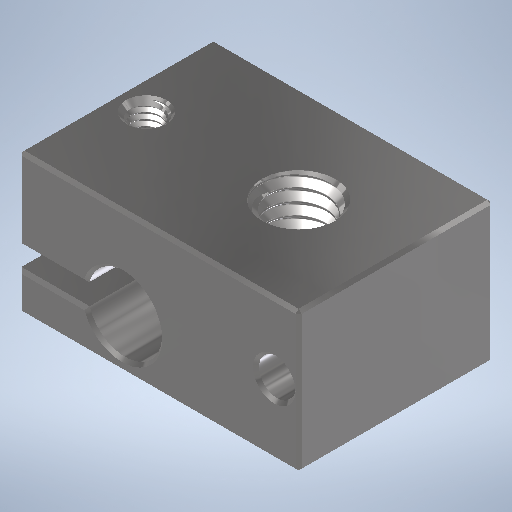
# Autodesk Inventor part: E3D-v6 Heater Block for Sensor Cartridges
Saved by Autodesk Inventor 2025.2 (Build 292293000, 293)
## iProperties
Created: 2018-03-24
Part Number: E3D-v6 Heater Block for Sensor Cartridges
Material: Aluminum 7075
Document SubType Name: Modeling
Designer: Samppa Turunen
Density: 2.81 g/cm^3
Appearance: Semi-Polished
Author: Samppa Turunen
Autodesk Inventor part; units mm, degrees
ref_plane "YZ Plane" through (0, 0, 0) normal (1, 0, 0) x (0, 1, 0)
ref_plane "XZ Plane" through (0, 0, 0) normal (0, 1, 0) x (-1, 0, 0)
ref_plane "XY Plane" through (0, 0, 0) normal (0, 0, 1) x (1, 0, 0)
sketch "Sketch1" plane through (0, 0, 0) normal (0, 1, 0) x (-1, 0, 0)
  line L0 (11.5, 8) -> (-11.5, 8)
  line L1 (-11.5, 8) -> (-11.5, -8)
  line L2 (-11.5, -8) -> (11.5, -8)
  line L3 (11.5, -8) -> (11.5, 8)
  line L4 (11.5, 8) -> (-11.5, -8) construction
  line L5 (-11.5, 8) -> (11.5, -8) construction
  point P0 (0, 0)
  dimension "d0" = 23
  dimension "d1" = 16
  constraints: 12 end point, 2 midpoint, 2 parallel, 1 horizontal, 1 perpendicular
  measures "d0" distance of L0.start L0.end
  measures "d1" distance of L1.end L0.end
extrude "Extrusion1" add sketch "Sketch1" along normal blind 11.5
sketch "Sketch2" plane through (0, 11.5, 0) normal (0, 1, 0) x (1, 0, 0)
  circle A0 centre (-9, 0) radius 1.5
  circle A1 centre (3.5, 0) radius 3
  point P0 (0, 0)
  dimension "d5" = 3
  dimension "d6" = 6
  constraints: 2 centre point
  measures "d5" diameter of A0
  measures "d6" diameter of A1
extrude "Extrusion2" cut sketch "Sketch2" against normal through all
sketch "Sketch3" plane through (-11.5, 0, 8) normal (0, 0, 1) x (1, 0, 0)
  circle A0 centre (21, 5.75) radius 1.5
  arc A1 (5.5872, 3.1) -> (5.5571, 4.7969) centre (8.5013, 4.0004) ccw
  line L0 (0, 3.1) -> (5.5872, 3.1)
  line L1 (0, 4.7969) -> (5.5571, 4.7969)
  line L2 (0, 3.1) -> (0, 4.7969)
  point P0 (11.5, 0)
  dimension "d9" = 3
  dimension "d10" = 6.1
  constraints: 6 end point, 2 centre point, 2 point on circle, 1 perpendicular
  measures "d9" diameter of A0
  measures "d10" diameter of A1
extrude "Extrusion3" cut sketch "Sketch3" along normal through all both and the other way through all
sketch "Sketch4" plane through (0, 0, 0) normal (0, -1, 0) x (1, 0, 0)
  circle A0 centre (9.5, 0) radius 1.5
  point P0 (0, 0)
  dimension "d13" = 3
  constraints: 1 centre point
  measures "d13" diameter of A0
extrude "Extrusion4" cut sketch "Sketch4" against normal up to next
sketch "Sketch6" plane through (3.5, 0, 0) normal (-1, 0, 0) x (0, 0, 1)
  line L0 (3.0474, 0) -> (3.0474, 11.5)
  line L1 (2.3474, 10.8) -> (2.3474, 0.7)
  line L2 (0, -2.3) -> (0, 13.8) projected
  line L3 (3.0474, 11.5) -> (2.3474, 10.8)
  line L4 (3.0474, 0) -> (2.3474, 0.7)
  dimension "d40" = 0.7
  constraints: 8 end point, 1 vertical
  measures "d40" distance between parallel lines of L0 L1
revolve "Revolution1" add sketch "Sketch6" angle 360 about axis through (3.5, 0, 0) along (0, 1, 0) separate body
sketch "Sketch5" plane through (3.5, 0, 3) normal (1, 0, 0) x (0, 1, 0)
  line L0 (-0.5925, -0.0535) -> (-0.5001, -0.0535) construction
  line L1 (0.0923, -0.5994) -> (-0.0001, -0.7595) construction
  line L2 (-1.0001, -0.7595) -> (-1.0925, -0.5994) construction
  line L3 (-0.4077, -0.0535) -> (-0.5001, 0.1066) construction
  line L4 (-0.5001, 0.1066) -> (-0.5925, -0.0535) construction
  line L5 (-1.0001, -0.7595) -> (-0.9077, -0.5994) construction
  line L6 (-0.4077, -0.0535) -> (-0.0925, -0.5994)
  line L7 (-1.0925, -0.5994) -> (-0.9077, -0.5994) construction
  arc A0 (-1.0925, -0.5994) -> (-1.0001, -0.6528) centre (-1.0001, -0.546) ccw construction
  line L8 (0.0923, -0.5994) -> (-0.0925, -0.5994) construction
  line L9 (-1.0001, -0.7595) -> (-1.0001, -0.5994) construction
  line L10 (-0.0001, -0.7595) -> (-0.0001, -0.5994) construction
  line L11 (-0.5001, 0.1066) -> (-0.5001, -0.0002) construction
  line L12 (-1.0001, -0.6528) -> (-0.0001, -0.6528)
  arc A1 (-1.0001, -0.6528) -> (-0.9077, -0.5994) centre (-1.0001, -0.546) ccw
  line L13 (-0.0925, -0.5994) -> (-0.0001, -0.7595) construction
  line L14 (-0.9077, -0.5994) -> (-0.5925, -0.0535)
  line L15 (-0.0001, -0.0002) -> (-0.0001, 0.0177)
  line L16 (-0.0001, 0.0177) -> (-0.0001, -0.0002)
  line L17 (-0.0001, -0.0002) -> (0.0334, -0.0002)
  arc A2 (-0.0925, -0.5994) -> (-0.0001, -0.6528) centre (-0.0001, -0.546) ccw
  arc A3 (-0.0001, -0.6528) -> (0.0923, -0.5994) centre (-0.0001, -0.546) ccw construction
  arc A4 (-0.5001, -0.0002) -> (-0.5925, -0.0535) centre (-0.5001, -0.1069) ccw
  arc A5 (-0.4077, -0.0535) -> (-0.5001, -0.0002) centre (-0.5001, -0.1069) ccw
  line L18 (-0.5001, -0.0002) -> (-0.5001, -0.0535) construction
  line L19 (-0.5001, -0.0535) -> (-0.4077, -0.0535) construction
  dimension "d22" = 60
  dimension "d23" = 0.1601
  dimension "d24" = 0.1601
  dimension "Sketch5_ThreadOffset" = 0
  dimension "Sketch5_MajorRadius" = 0.6526
  dimension "d27" = 1
  dimension "Sketch5_MinorRadius" = 0
  constraints: 40 end point, 12 point on circle, 10 parallel, 8 tangent, 6 centre point, 6 collinear, 2 midpoint, 2 point on line, 1 horizontal, 1 perpendicular, 3 other
  measures "d22" angle of L6 L14
  measures "d23" distance of L3.end L0.end
  measures "d24" distance of L1.end L10.end
  measures "Sketch5_ThreadOffset" distance between parallel lines of L15 L10
  measures "Sketch5_MajorRadius" distance from line of L12 L15.start
  measures "d27" distance from line of L1.end L9
  measures "Sketch5_MinorRadius" distance edge to line of A5 L17
coil "Coil1" sketch "Sketch5" operation cut axis through (3.5, 0, 0) along (0, 1, 0) pitch 1.001 turns 13.486513 hand right bodies 2
sketch "Sketch8" plane through (-9, 4.7969, 0) normal (-1, 0, 0) x (0, 0, 1)
  line L0 (1.6737, 0) -> (1.6737, 6.7031)
  line L1 (1.1737, 6.2031) -> (1.1737, 0)
  line L2 (1.1737, 0) -> (1.6737, 0)
  line L3 (0, -1.3406) -> (0, 8.0438) projected
  line L4 (1.6737, 6.7031) -> (1.1737, 6.2031)
  dimension "d60" = 0.5
  dimension "d62" = 45
  constraints: 8 end point, 1 vertical
  measures "d60" distance between parallel lines of L0 L1
  measures "d62" angle of L0 L4
revolve "Revolution2" add sketch "Sketch8" angle 360 about axis through (-9, 4.7969, 0) along (0, 1, 0) separate body
chamfer "Chamfer2" distance 0.047 angle 45 2 edges at (3.5, 0, -3.0474) (3.5, 11.5, -3.0474)
sketch "Sketch7" plane through (-9, 4.7969, 1.5) normal (1, 0, 0) x (0, 1, 0)
  line L0 (-0.2963, -0.0268) -> (-0.2501, -0.0268) construction
  line L1 (0.0461, -0.2998) -> (-0.0001, -0.3798) construction
  line L2 (-0.5001, -0.3798) -> (-0.5463, -0.2998) construction
  line L3 (-0.2039, -0.0268) -> (-0.2501, 0.0532) construction
  line L4 (-0.2501, 0.0532) -> (-0.2963, -0.0268) construction
  line L5 (-0.5001, -0.3798) -> (-0.4539, -0.2998) construction
  line L6 (-0.2039, -0.0268) -> (-0.0463, -0.2998)
  line L7 (-0.5463, -0.2998) -> (-0.4539, -0.2998) construction
  arc A0 (-0.5463, -0.2998) -> (-0.5001, -0.3265) centre (-0.5001, -0.2731) ccw construction
  line L8 (0.0461, -0.2998) -> (-0.0463, -0.2998) construction
  line L9 (-0.5001, -0.3798) -> (-0.5001, -0.2998) construction
  line L10 (-0.0001, -0.3798) -> (-0.0001, -0.2998) construction
  line L11 (-0.2501, 0.0532) -> (-0.2501, -0.0002) construction
  line L12 (-0.5001, -0.3265) -> (-0.0001, -0.3265)
  arc A1 (-0.5001, -0.3265) -> (-0.4539, -0.2998) centre (-0.5001, -0.2731) ccw
  line L13 (-0.0463, -0.2998) -> (-0.0001, -0.3798) construction
  line L14 (-0.4539, -0.2998) -> (-0.2963, -0.0268)
  line L15 (-0.0001, -0.0002) -> (-0.0001, 0.0177)
  line L16 (-0.0001, 0.0177) -> (-0.0001, -0.0002)
  line L17 (-0.0001, -0.0002) -> (0.0334, -0.0002)
  arc A2 (-0.0463, -0.2998) -> (-0.0001, -0.3265) centre (-0.0001, -0.2731) ccw
  arc A3 (-0.0001, -0.3265) -> (0.0461, -0.2998) centre (-0.0001, -0.2731) ccw construction
  arc A4 (-0.2501, -0.0002) -> (-0.2963, -0.0268) centre (-0.2501, -0.0535) ccw
  arc A5 (-0.2039, -0.0268) -> (-0.2501, -0.0002) centre (-0.2501, -0.0535) ccw
  line L18 (-0.2501, -0.0002) -> (-0.2501, -0.0268) construction
  line L19 (-0.2501, -0.0268) -> (-0.2039, -0.0268) construction
  dimension "d42" = 60
  dimension "d43" = 0.08
  dimension "d44" = 0.08
  dimension "Sketch7_ThreadOffset" = 0
  dimension "Sketch7_MajorRadius" = 0.3263
  dimension "d47" = 0.5
  dimension "Sketch7_MinorRadius" = 0
  constraints: 40 end point, 12 point on circle, 10 parallel, 8 tangent, 6 centre point, 6 collinear, 2 midpoint, 2 point on line, 1 horizontal, 1 perpendicular, 3 other
  measures "d42" angle of L6 L14
  measures "d43" distance of L3.end L0.end
  measures "d44" distance of L1.end L10.end
  measures "Sketch7_ThreadOffset" distance between parallel lines of L15 L10
  measures "Sketch7_MajorRadius" distance from line of L12 L15.start
  measures "d47" distance from line of L1.end L9
  measures "Sketch7_MinorRadius" distance edge to line of A5 L17
coil "Coil2" sketch "Sketch7" operation cut axis through (-9, 4.7969, 0) along (0, 1, 0) pitch 0.5005 turns 15.390901 hand right bodies 3
sketch "Sketch10" plane through (9.5, 5.75, 0) normal (1, 0, 0) x (0, 0, 1)
  line L0 (1.6737, 0) -> (1.6737, 5.75)
  line L1 (1.1737, 5.25) -> (1.1737, 0)
  line L2 (1.1737, 0) -> (1.6737, 0)
  line L3 (0, -1.15) -> (0, 6.9) projected
  line L4 (1.6737, 5.75) -> (1.1737, 5.25)
  line L5 (1.6737, 5.75) -> (2.3808, 5.75) construction
  line L6 (-1.5, 5.75) -> (1.5, 5.75) projected
  dimension "d81" = 0.5
  dimension "d82" = 135
  dimension "d92" = 5.75
  constraints: 10 end point, 1 equal length, 1 horizontal, 1 vertical
  measures "d81" distance between parallel lines of L0 L1
  measures "d82" angle of L4 L5
  measures "d92" distance between parallel lines of L6 L2
revolve "Revolution3" add sketch "Sketch10" angle 360 about axis through (9.5, 5.75, 0) along (0, -1, 0) separate body
sketch "Sketch13" plane through (-11.5, 0, 8) normal (0, 0, 1) x (1, 0, 0)
  circle A0 centre (21, 5.75) radius 1.5 projected
  circle A1 centre (21, 5.75) radius 1.5
  line L0 (22.5, 0) -> (22.5, 5.75) projected
  point P0 (11.5, 0)
  constraints: 1 centre point, 1 coincident, 1 horizontal alignment, 1 tangent
extrude "Extrusion5" cut sketch "Sketch13" against normal through all bodies 1 2 4
sketch "Sketch9" plane through (9.5, 5.75, 1.5) normal (-1, 0, 0) x (0, -1, 0)
  line L0 (-0.2963, -0.0268) -> (-0.2501, -0.0268) construction
  line L1 (0.0461, -0.2998) -> (-0.0001, -0.3798) construction
  line L2 (-0.5001, -0.3798) -> (-0.5463, -0.2998) construction
  line L3 (-0.2039, -0.0268) -> (-0.2501, 0.0532) construction
  line L4 (-0.2501, 0.0532) -> (-0.2963, -0.0268) construction
  line L5 (-0.5001, -0.3798) -> (-0.4539, -0.2998) construction
  line L6 (-0.2039, -0.0268) -> (-0.0463, -0.2998)
  line L7 (-0.5463, -0.2998) -> (-0.4539, -0.2998) construction
  arc A0 (-0.5463, -0.2998) -> (-0.5001, -0.3265) centre (-0.5001, -0.2731) ccw construction
  line L8 (0.0461, -0.2998) -> (-0.0463, -0.2998) construction
  line L9 (-0.5001, -0.3798) -> (-0.5001, -0.2998) construction
  line L10 (-0.0001, -0.3798) -> (-0.0001, -0.2998) construction
  line L11 (-0.2501, 0.0532) -> (-0.2501, -0.0002) construction
  line L12 (-0.5001, -0.3265) -> (-0.0001, -0.3265)
  arc A1 (-0.5001, -0.3265) -> (-0.4539, -0.2998) centre (-0.5001, -0.2731) ccw
  line L13 (-0.0463, -0.2998) -> (-0.0001, -0.3798) construction
  line L14 (-0.4539, -0.2998) -> (-0.2963, -0.0268)
  line L15 (-0.0001, -0.0002) -> (-0.0001, 0.0177)
  line L16 (-0.0001, 0.0177) -> (-0.0001, -0.0002)
  line L17 (-0.0001, -0.0002) -> (0.0334, -0.0002)
  arc A2 (-0.0463, -0.2998) -> (-0.0001, -0.3265) centre (-0.0001, -0.2731) ccw
  arc A3 (-0.0001, -0.3265) -> (0.0461, -0.2998) centre (-0.0001, -0.2731) ccw construction
  arc A4 (-0.2501, -0.0002) -> (-0.2963, -0.0268) centre (-0.2501, -0.0535) ccw
  arc A5 (-0.2039, -0.0268) -> (-0.2501, -0.0002) centre (-0.2501, -0.0535) ccw
  line L18 (-0.2501, -0.0002) -> (-0.2501, -0.0268) construction
  line L19 (-0.2501, -0.0268) -> (-0.2039, -0.0268) construction
  dimension "d63" = 60
  dimension "d64" = 0.08
  dimension "d65" = 0.08
  dimension "Sketch9_ThreadOffset" = 0
  dimension "Sketch9_MajorRadius" = 0.3263
  dimension "d68" = 0.5
  dimension "Sketch9_MinorRadius" = 0
  constraints: 40 end point, 12 point on circle, 10 parallel, 8 tangent, 6 centre point, 6 collinear, 2 midpoint, 2 point on line, 1 horizontal, 1 perpendicular, 3 other
  measures "d63" angle of L6 L14
  measures "d64" distance of L3.end L0.end
  measures "d65" distance of L1.end L10.end
  measures "Sketch9_ThreadOffset" distance between parallel lines of L15 L10
  measures "Sketch9_MajorRadius" distance from line of L12 L15.start
  measures "d68" distance from line of L1.end L9
  measures "Sketch9_MinorRadius" distance edge to line of A5 L17
coil "Coil3" sketch "Sketch9" operation cut axis through (9.5, 5.75, 0) along (0, -1, 0) pitch 0.5005 turns 13.486513 hand right bodies 4
chamfer "Chamfer1" distance 0.174 angle 45 2 edges at (8, 0, 0) (-10.5, 11.5, 0)
chamfer "Chamfer3" distance 0.25 angle 45 20 edges at (0, 11.5, 8) (11.5, 5.75, 8) (11.5, 11.5, 0) (-11.5, 11.5, 0) (-11.5, 8.1484, 8) (-11.5, 1.55, 8) (0, 0, 8) (11.5, 5.75, -8) (11.5, 0, 0) (0, 0, -8) (0, 11.5, -8) (-11.5, 8.1484, -8) (0.0508, 4.0545, -8) (8, 5.75, -8) (-8.7064, 3.1, -8) (-8.7214, 4.7969, -8) (-8.7214, 4.7969, 8) (-8.7064, 3.1, 8) (0.0508, 4.0545, 8) (8, 5.75, 8)
equation "\"d22\" = d29"
equation "\"d23\" = 0.160083 * Sketch5_Pitch"
equation "\"d24\" = 0.160083 * Sketch5_Pitch"
equation "\"d27\" = Sketch5_Pitch"
equation "\"d42\" = d49"
equation "\"d43\" = 0.160083 * Sketch7_Pitch"
equation "\"d44\" = 0.160083 * Sketch7_Pitch"
equation "\"d47\" = Sketch7_Pitch"
equation "\"d63\" = d70"
equation "\"d64\" = 0.160083 * Sketch9_Pitch"
equation "\"d65\" = 0.160083 * Sketch9_Pitch"
equation "\"d68\" = Sketch9_Pitch"
equation "\"d29\" = 60deg"
equation "\"Sketch5_Pitch\" = 1"
equation "\"d49\" = 60deg"
equation "\"Sketch7_Pitch\" = 0.5"
equation "\"d70\" = 60deg"
equation "\"Sketch9_Pitch\" = 0.5"
body "Solid1"
body "Solid2"
body "Solid3"
body "Solid4"
